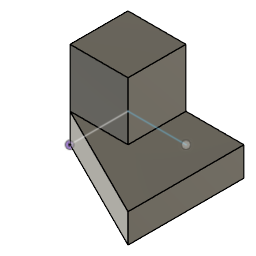
Ex3-lab1 (Autodesk Fusion 360 design; units mm, degrees)
part number: 2026-03-02-19-50-49-763
Autodesk Fusion 360 part; units mm, degrees
sketch "Sketch1" plane through (0, 0, 0) normal (0, 0, 1) x (1, 0, 0)
  line L0 (0, 0) -> (0, 20)
  line L1 (0, 20) -> (40, 20)
  line L2 (40, 20) -> (40, -20)
  line L3 (40, -20) -> (0, 0)
  line L4 (0, 0) -> (20, 0)
  line L5 (20, 0) -> (20, 20)
  dimension "d1" = 20
  dimension "d2" = 40
  dimension "d3" = 40
  dimension "d4" = 20
  constraint coincident L0.start L3.end
  constraint vertical L0
  constraint perpendicular L0 L1
  constraint perpendicular L1 L2
  constraint perpendicular L0 L4
  constraint midpoint L1 L5.end
  measures "d1" distance of L0.start L0.end
  measures "d2" distance of L0.end L1.end
  measures "d3" distance of L1.end L2.end
  measures "d4" distance of L0.start L4.end
extrude "Extrude1" add sketch "Sketch1" along normal blind 10 contours L1 L2 L3 L4 L5
sketch "Sketch2" plane through (0, 0, 0) normal (0, 0, 1) x (1, 0, 0)
  line L0 (0, 0) -> (0, 20)
  line L1 (0, 20) -> (20, 20)
  constraint coincident L0.start origin
  constraint vertical L0
  constraint perpendicular L0 L1
sketch "Sketch3" plane through (0, 0, 0) normal (0, 0, 1) x (1, 0, 0)
sketch "Sketch4" plane through (0, 0, 0) normal (0, 0, 1) x (1, 0, 0)
  line L0 (20, 20) -> (0, 20)
  line L1 (0, 20) -> (0, 0)
  line L2 (0, 0) -> (20, 0)
  line L3 (20, 0) -> (20, 20)
  constraint horizontal L0
  constraint coincident L1.end L2.start
  constraint perpendicular L0 L1
  constraint perpendicular L1 L2
  constraint perpendicular L0 L3
extrude "Extrude2" add sketch "Sketch4" along normal blind 30
